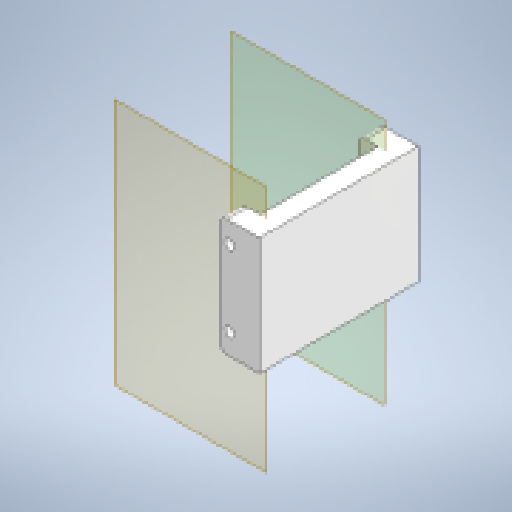
# Autodesk Inventor part: 3
Saved by Autodesk Inventor 2024.3 (Build 283343000, 343)
## iProperties
Created: 2024-09-05
Part Number: 3
Material: LCP 플라스틱
Document SubType Name: Modeling
Designer: 구지현
Density: 1.626 g/cm^3
Appearance: 매끄러움 - 흰색
Author: 구지현
Autodesk Inventor part; units mm, degrees
ref_plane "YZ Plane" through (0, 0, 0) normal (1, 0, 0) x (0, 1, 0)
ref_plane "XZ Plane" through (0, 0, 0) normal (0, 1, 0) x (-1, 0, 0)
ref_plane "XY Plane" through (0, 0, 0) normal (0, 0, 1) x (1, 0, 0)
ref_plane "작업 평면1" through (0, 0, 0) normal (0, 0, 1) x (1, 0, 0)
sketch "스케치1" plane through (0, 0, 0) normal (0, 0, 1) x (1, 0, 0)
  circle A0 centre (0, 0) radius 1.5 projected
  circle A1 centre (0, 0) radius 4.9 projected
  circle A2 centre (0, 0) radius 7.05 projected
  circle A3 centre (7.7781, 7.7783) radius 1.55 projected
  circle A4 centre (-7.7783, 7.7781) radius 1.55 projected
  circle A5 centre (-7.7781, -7.7783) radius 1.55 projected
  circle A6 centre (7.7783, -7.7781) radius 1.55 projected
  circle A7 centre (0, 0) radius 5 projected
  circle A8 centre (0, 0) radius 13.9 projected
  circle A9 centre (0.0001, -11) radius 1.55 projected
  circle A10 centre (-11, -0.0001) radius 1.55 projected
  circle A11 centre (-0.0001, 11) radius 1.55 projected
  circle A12 centre (11, 0.0001) radius 1.55 projected
  line L0 (0, 0) -> (-50, 0)
  line L1 (-15, 14.5) -> (-11.5, 14.5) projected
  line L2 (-15, 14.5) -> (-20.1, 8.5) projected
  line L3 (-20.1, 8.5) -> (-20.1, -44.6) projected
  line L4 (-20.1, -44.6) -> (-15, -50.6) projected
  line L5 (-15, -50.6) -> (15, -50.6) projected
  line L6 (15, -50.6) -> (20.1, -44.6) projected
  line L7 (20.1, -44.6) -> (20.1, 8.5) projected
  line L8 (20.1, 8.5) -> (15, 14.5) projected
  line L9 (11.5, 14.5) -> (15, 14.5) projected
  arc A13 (14.5, 11.5) -> (11.5, 14.5) centre (11.5, 11.5) ccw projected
  line L10 (14.5, -42) -> (14.5, 11.5) projected
  arc A14 (11.5, -45) -> (14.5, -42) centre (11.5, -42) ccw projected
  line L11 (-11.5, -45) -> (11.5, -45) projected
  arc A15 (-14.5, -42) -> (-11.5, -45) centre (-11.5, -42) ccw projected
  line L12 (-14.5, 11.5) -> (-14.5, -42) projected
  arc A16 (-11.5, 14.5) -> (-14.5, 11.5) centre (-11.5, 11.5) ccw projected
  circle A17 centre (17.3, 4) radius 1.35 projected
  circle A18 centre (17.3, -18) radius 1.35 projected
  circle A19 centre (17.3, -40) radius 1.35 projected
  circle A20 centre (11, -47.8) radius 1.35 projected
  circle A21 centre (-17.3, 4) radius 1.35 projected
  circle A22 centre (-17.3, -18) radius 1.35 projected
  circle A23 centre (-17.3, -40) radius 1.35 projected
  circle A24 centre (-11, -47.8) radius 1.35 projected
  circle A25 centre (-17.3, -18) radius 1.45
  circle A26 centre (-17.3, 4) radius 1.45
  arc A27 (-14.6, -42) -> (-11.5, -45.1) centre (-11.5, -42) ccw
  line L13 (-11.5, -45.1) -> (11.5, -45.1)
  arc A28 (11.5, -45.1) -> (14.6, -42) centre (11.5, -42) ccw
  line L14 (14.6, -22) -> (14.6, 8)
  arc A29 (14.6, 11.5) -> (12.5954, 14.4) centre (11.5, 11.5) ccw
  line L15 (12.5954, 14.4) -> (14.9538, 14.4)
  line L16 (14.9538, 14.4) -> (18.6938, 10)
  line L17 (20, -24) -> (20, -44.5632)
  line L18 (20, -44.5632) -> (14.9538, -50.5)
  line L19 (14.9538, -50.5) -> (-14.9538, -50.5)
  line L20 (-14.9538, -50.5) -> (-20, -44.5632)
  line L21 (-18.6938, 10) -> (-14.9538, 14.4)
  line L22 (-14.9538, 14.4) -> (-12.5954, 14.4)
  arc A30 (-12.5954, 14.4) -> (-14.6, 11.5) centre (-11.5, 11.5) ccw
  line L23 (-14.6, 11.5) -> (-14.6, -42)
  line L24 (-17.3, 4) -> (-17.3, 10)
  line L25 (-14.6, 10) -> (-18.0941, 10)
  line L26 (-17.3, -19.35) -> (-17.3, -24)
  line L27 (-14.6, -24) -> (-18.0059, -24)
  line L28 (-20, -44.5632) -> (-20, -24)
  line L29 (-20.0059, -22.0059) -> (-20.0941, 7.9941)
  arc A31 (-18.0941, 10) -> (-20.0941, 7.9941) centre (-18.0941, 8) ccw
  arc A32 (-20.0059, -22.0059) -> (-18.0059, -24) centre (-18.0059, -22) ccw
  line L30 (-36.7788, 11.5) -> (-35.2788, 11.5) projected
  line L31 (-36.7788, 11.5) -> (-36.7788, -41.5) projected
  line L32 (-35.2788, -41.5) -> (-36.7788, -41.5) projected
  spline S0 degree 3 poles (-34.7788, -41) (-34.788, -41.241) (-35.0376, -41.5) (-35.2788, -41.5) knots 0 0 0 0 1 1 1 1 projected
  line L33 (-34.7788, 11) -> (-34.7788, -41) projected
  ellipse E0 centre (-35.2788, 11) end of major axis (-35.2788, 11.5) minor radius 0.5 (-34.7788, 11) -> (-35.2788, 11.5) ccw projected
  line L34 (16.6, -24) -> (18.1, -24)
  line L35 (16.6, 10) -> (18.1, 10)
  line L36 (20.1, -22) -> (20.1, 8)
  circle A33 centre (17.3, 4) radius 1.45
  circle A34 centre (17.3, -18) radius 1.45
  line L37 (18.1, -24) -> (20.1, -24)
  line L38 (20.1, -24) -> (20.1, -22)
  arc A35 (14.6, -22) -> (16.6, -24) centre (16.6, -22) ccw
  line L39 (20.1, 8) -> (20.1, 10)
  line L40 (18.1, 10) -> (20.1, 10)
  arc A36 (16.6, 10) -> (14.6, 8) centre (16.6, 8) ccw
  point P0 (0, 0)
  point P1 (-20.1, 10)
  point P2 (-20.1, -24)
  point P3 (14.6, -24)
  point P4 (14.6, 10)
  point P5 (-19.9941, 8.6246)
  point P6 (-19.0167, 9.7745)
  point P7 (18.825, 10)
  point P8 (20.1, 8.5)
  dimension "d0" = 50
  dimension "d1" = 0.1
  dimension "d2" = 0.1
  dimension "d3" = 0.1
  dimension "d4" = 6
  dimension "d5" = 6
  dimension "d6" = 2
  dimension "d10" = 0.1
  dimension "d11" = 0.1
  dimension "d12" = 2
  dimension "d13" = 2
  constraints: 50 end point, 19 point on line, 16 point on circle, 12 centre point, 8 tangent, 4 horizontal, 3 perpendicular, 3 vertical, 1 collinear, 1 equal radius, 1 vertical alignment, 11 other
  measures "d0" distance of L0.start L0.end
  measures "d2" radial gap between concentric circles of A21 A26
  measures "d3" distance between parallel lines of L12 L23
  measures "d4" distance of L24.start L24.end
  measures "d5" distance of A25.centre L26.end
  measures "d6" radius of A31
  measures "d10" radial gap between concentric circles of A17 A33
  measures "d11" radial gap between concentric circles of A18 A34
  measures "d12" radius of A35
  measures "d13" radius of A36
extrude "돌출1" add sketch "스케치1" along normal blind 6 contours L37 L34 A35 L14 A36 L35 L40 L8 L7 | L40 L39 L8
ref_plane "작업 평면2" through (0, 0, -34) normal (0, 0, -1) x (-1, 0, 0)
sketch "스케치2" plane through (0, 0, -34) normal (0, 0, -1) x (-1, 0, 0)
  line L0 (-16.6, -24) -> (-20.1, -24) projected
  line L1 (-20.1, -24) -> (-20.1, 10) projected
  line L2 (-20.1, 10) -> (-16.6, 10) projected
  arc A0 (-14.6, 8) -> (-16.6, 10) centre (-16.6, 8) ccw projected
  line L3 (-14.6, 8) -> (-14.6, -22) projected
  arc A1 (-16.6, -24) -> (-14.6, -22) centre (-16.6, -22) ccw projected
  circle A2 centre (-17.3, 4) radius 1.45 projected
  circle A3 centre (-17.3, -18) radius 1.45 projected
  point P0 (0, 0)
extrude "돌출2" add sketch "스케치2" along normal blind 6
sketch "스케치3" plane through (20.1, -24, -34) normal (1, 0, 0) x (0, 0, -1)
  line L0 (0, 34) -> (0, 0) projected
  line L1 (0, 0) -> (6, 0) projected
  line L2 (6, 34) -> (6, 0) projected
  line L3 (0, 34) -> (6, 34) projected
  line L4 (-34, 0) -> (-34, 34) projected
  line L5 (-34, 34) -> (-40, 34) projected
  line L6 (-40, 0) -> (-40, 34) projected
  line L7 (-34, 0) -> (-40, 0) projected
  line L8 (6, 0) -> (-40, 0)
  line L9 (-40, 0) -> (-40, 34)
  line L10 (-40, 34) -> (6, 34)
  line L11 (6, 34) -> (6, 0)
  point P0 (-34, 24)
  constraints: 8 end point, 2 parallel, 1 horizontal, 1 perpendicular
extrude "돌출3" add sketch "스케치3" along normal blind 5.901
sketch "스케치4" plane through (26.001, -24, -34) normal (1, 0, 0) x (0, 0, -1)
  line L0 (-5.3426, 23.9933) -> (-5.3329, 43.9933) projected
  line L1 (-5.3329, 43.9933) -> (-32.9329, 44.0067) projected
  line L2 (-32.9329, 44.0067) -> (-32.9426, 24.0067) projected
  arc A0 (-32.9426, 24.0067) -> (-5.3426, 23.9933) centre (-19.1426, 24) ccw projected
  circle A1 centre (-11.3683, 16.218) radius 1.65 projected
  circle A2 centre (-19.148, 13) radius 1.65 projected
  circle A3 centre (-26.9246, 16.2256) radius 1.65 projected
  circle A4 centre (-30.1426, 24.0054) radius 1.65 projected
  circle A5 centre (-26.917, 31.782) radius 1.65 projected
  circle A6 centre (-19.1373, 35) radius 1.65 projected
  circle A7 centre (-11.3607, 31.7744) radius 1.65 projected
  circle A8 centre (-8.1426, 23.9946) radius 1.65 projected
  circle A9 centre (-19.1426, 24) radius 5.1 projected
  circle A10 centre (-19.1426, 24) radius 4.1
  point P0 (-34, 24)
  dimension "d26" = 8.2
  constraints: 1 centre point, 1 coincident
  measures "d26" diameter of A10
extrude "돌출4" cut sketch "스케치4" against normal blind 3 contours A10
sketch "스케치6" plane through (26.001, -24, -34) normal (1, 0, 0) x (0, 0, -1)
  line L0 (-5.3426, 23.9933) -> (-5.3329, 43.9933) projected
  line L1 (-5.3329, 43.9933) -> (-32.9329, 44.0067) projected
  line L2 (-32.9329, 44.0067) -> (-32.9426, 24.0067) projected
  arc A0 (-32.9426, 24.0067) -> (-5.3426, 23.9933) centre (-19.1426, 24) ccw projected
  circle A1 centre (-11.3683, 16.218) radius 1.65 projected
  circle A2 centre (-19.148, 13) radius 1.65 projected
  circle A3 centre (-26.9246, 16.2256) radius 1.65 projected
  circle A4 centre (-30.1426, 24.0054) radius 1.65 projected
  circle A5 centre (-26.917, 31.782) radius 1.65 projected
  circle A6 centre (-19.1373, 35) radius 1.65 projected
  circle A7 centre (-11.3607, 31.7744) radius 1.65 projected
  circle A8 centre (-8.1426, 23.9946) radius 1.65 projected
  circle A9 centre (-19.1426, 24) radius 5.1 projected
  circle A10 centre (-19.1426, 24) radius 3.55
  circle A11 centre (-19.1426, 24) radius 4.1
  point P0 (-34, 24)
  dimension "d27" = 7.1
  dimension "d28" = 8.2
  constraints: 2 centre point, 2 coincident
  measures "d27" diameter of A10
  measures "d28" diameter of A11
extrude "돌출6" add sketch "스케치6" against normal blind 2.2 contours A9 | A11
sketch "스케치7" plane through (16.6, -24, 0) normal (0, -1, 0) x (1, 0, 0)
  line L0 (0, 0) -> (3.5, 0) projected
  line L1 (3.5, 0) -> (3.5, -34) projected
  line L2 (3.5, -34) -> (0, -34) projected
  line L3 (0, -34) -> (0, -40) projected
  line L4 (0, -40) -> (9.401, -40) projected
  line L5 (9.401, 6) -> (9.401, -40) projected
  line L6 (0, 6) -> (9.401, 6) projected
  line L7 (0, 0) -> (0, 6) projected
  line L8 (0, -34) -> (-2, -34) projected
  line L9 (-2, -34) -> (-2, -40) projected
  line L10 (0, -40) -> (-2, -40) projected
  line L11 (0, -34) -> (0, -40) projected
  line L12 (-2, 0) -> (0, 0) projected
  line L13 (0, 0) -> (0, 6) projected
  line L14 (-2, 6) -> (0, 6) projected
  line L15 (-2, 0) -> (-2, 6) projected
  line L16 (3.6, -34.1) -> (3.6, 0.1)
  line L17 (3.6, 0.1) -> (0.1, 0.1)
  line L18 (0.1, 0.1) -> (0.1, 5.9)
  line L19 (0.1, 5.9) -> (9.301, 5.9)
  line L20 (9.301, 5.9) -> (9.301, -39.9)
  line L21 (9.301, -39.9) -> (0.1, -39.9)
  line L22 (0.1, -39.9) -> (0.1, -34.1)
  line L23 (0.1, -34.1) -> (3.6, -34.1)
  line L24 (-0.1, 0.1) -> (-1.9, 0.1)
  line L25 (-1.9, 0.1) -> (-1.9, 5.9)
  line L26 (-1.9, 5.9) -> (-0.1, 5.9)
  line L27 (-0.1, 5.9) -> (-0.1, 0.1)
  line L28 (-1.9, -34.1) -> (-0.1, -34.1)
  line L29 (-0.1, -34.1) -> (-0.1, -39.9)
  line L30 (-0.1, -39.9) -> (-1.9, -39.9)
  line L31 (-1.9, -39.9) -> (-1.9, -34.1)
  line L32 (3.6, -34.1) -> (3.6, 0.1)
  line L33 (3.6, 0.1) -> (-2, 0.1)
  line L34 (-2, 0.1) -> (-2, -34.1)
  line L35 (-2, -34.1) -> (3.6, -34.1)
  point P0 (-16.6, 0)
  point P1 (-1.9, 0.1)
  point P2 (-2, 0.1)
  point P3 (-2, -34.1)
  point P4 (0.1, -34.1)
  point P5 (0.1, 0.1)
  point P6 (-0.1, 0.1)
  dimension "d31" = 0.1
  dimension "d32" = 0.1
  dimension "d33" = 0.1
  constraints: 40 end point, 3 equal length, 1 perpendicular, 13 other
  measures "d31" distance between parallel lines of L1 L16
  measures "d32" distance between parallel lines of L12 L24
  measures "d33" distance between parallel lines of L8 L28
extrude "돌출7" cut sketch "스케치7" against normal through all contours L7 L33 L17 L16 L23 L35 L3 L2 L1 L0 | L12 L15 L33 L24 L7 | L0 L1 L2 L8 L34 L12 | L8 L3 L35 L28 L9
sketch "스케치8" plane through (26.001, -24, -34) normal (1, 0, 0) x (0, 0, -1)
  circle A0 centre (-19.1426, 24) radius 3.55
  line L0 (6, 34) -> (-40, 34) projected
  line L1 (-40, 34) -> (-40, 0) projected
  line L2 (-40, 0) -> (6, 0) projected
  line L3 (6, 0) -> (6, 34) projected
  line L4 (-34, -20.6) -> (-34, 32.5) projected
  line L5 (0, -20.6) -> (0, 32.5) projected
  circle A1 centre (-19.1426, 24) radius 3.55 projected
  circle A2 centre (-18.5217, 13.1058) radius 1.55 projected
  circle A3 centre (-6.1058, 22.4783) radius 1.55 projected
  circle A4 centre (-15.4783, 34.8942) radius 1.55 projected
  circle A5 centre (-27.8942, 25.5217) radius 1.55 projected
  circle A6 centre (-17, 24) radius 5 projected
  circle A7 centre (-17, 24) radius 13.9 projected
  circle A8 centre (-23.6274, 32.7794) radius 1.55 projected
  circle A9 centre (-8.2206, 30.6274) radius 1.55 projected
  circle A10 centre (-10.3726, 15.2206) radius 1.55 projected
  circle A11 centre (-25.7794, 17.3726) radius 1.55 projected
  circle A12 centre (-17, 24) radius 1.55
  dimension "d44" = 3.1
  constraints: 2 centre point, 1 coincident
  measures "d44" diameter of A12
extrude "돌출8" cut sketch "스케치8" against normal through all contours A0 A12 | A0 A12
sketch "스케치9" plane through (26.001, -24, -34) normal (1, 0, 0) x (0, 0, -1)
  line L0 (6, 34) -> (-40, 34) projected
  line L1 (-40, 34) -> (-40, 0) projected
  line L2 (-40, 0) -> (6, 0) projected
  line L3 (6, 0) -> (6, 34) projected
  arc A0 (-15.6911, 24.8302) -> (-15.6911, 23.1698) centre (-19.1426, 24) ccw projected
  line L4 (0.1, 34) -> (-34.1, 34) projected
  line L5 (0.1, 0) -> (0.1, 34) projected
  line L6 (-34.1, 0) -> (0.1, 0) projected
  line L7 (-34.1, 0) -> (-34.1, 34) projected
  arc A1 (-15.6911, 23.1698) -> (-15.6911, 24.8302) centre (-17, 24) ccw projected
  point P0 (-34, 24)
extrude "돌출9" add sketch "스케치9" against normal up to surface (5.801 mm away) contours A1 A0
sketch "스케치10" plane through (26.001, -24, -34) normal (1, 0, 0) x (0, 0, -1)
  line L0 (6, 34) -> (-40, 34) projected
  line L1 (-40, 34) -> (-40, 0) projected
  line L2 (-40, 0) -> (6, 0) projected
  line L3 (6, 0) -> (6, 34) projected
  circle A0 centre (-17, 24) radius 4
  point P0 (-34, 24)
  dimension "d41" = 8
  constraints: 1 centre point
  measures "d41" diameter of A0
extrude "돌출10" add sketch "스케치10" against normal up to surface (5.801 mm away) contours A0
sketch "스케치11" plane through (26.001, -24, -34) normal (1, 0, 0) x (0, 0, -1)
  circle A0 centre (-18.5217, 13.1058) radius 1.55 projected
  circle A1 centre (-6.1058, 22.4783) radius 1.55 projected
  circle A2 centre (-15.4783, 34.8942) radius 1.55 projected
  circle A3 centre (-27.8942, 25.5217) radius 1.55 projected
  circle A4 centre (-17, 24) radius 5 projected
  circle A5 centre (-17, 24) radius 13.9 projected
  circle A6 centre (-23.6274, 32.7794) radius 1.55 projected
  circle A7 centre (-8.2206, 30.6274) radius 1.55 projected
  circle A8 centre (-10.3726, 15.2206) radius 1.55 projected
  circle A9 centre (-25.7794, 17.3726) radius 1.55 projected
  circle A10 centre (-17, 24) radius 1.6
  point P0 (-34, 24)
  dimension "d45" = 3.2
  constraints: 1 centre point, 1 coincident
  measures "d45" diameter of A10
extrude "돌출11" cut sketch "스케치11" against normal blind 10 contours A10
